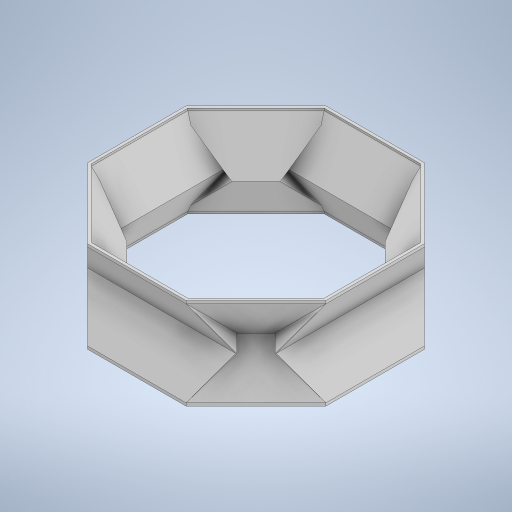
# Autodesk Inventor part: 팔각형 OV-PAM 층 한개
Saved by Autodesk Inventor 2024 (Build 280153000, 153)
## iProperties
Created: 2023-06-16
Part Number: 팔각형 OV-PAM 층 한개
Material: 일반
Document SubType Name: Modeling
Designer: jsw
Density: 1 g/cm^3
Appearance: 기본값
Author: jsw
Autodesk Inventor part; units mm, degrees
ref_plane "YZ Plane" through (0, 0, 0) normal (1, 0, 0) x (0, 1, 0)
ref_plane "XZ Plane" through (0, 0, 0) normal (0, 1, 0) x (-1, 0, 0)
ref_plane "XY Plane" through (0, 0, 0) normal (0, 0, 1) x (1, 0, 0)
sketch "스케치1" plane through (0, 0, 0) normal (0, 1, 0) x (-1, 0, 0)
  line L0 (-32.591883, 13.5) -> (-13.5, 32.591883)
  line L1 (-13.5, 32.591883) -> (13.5, 32.591883)
  line L2 (13.5, 32.591883) -> (32.591883, 13.5)
  line L3 (32.591883, 13.5) -> (32.591883, -13.5)
  line L4 (32.591883, -13.5) -> (13.5, -32.591883)
  line L5 (13.5, -32.591883) -> (-13.5, -32.591883)
  line L6 (-13.5, -32.591883) -> (-32.591883, -13.5)
  line L7 (-32.591883, -13.5) -> (-32.591883, 13.5)
  line L8 (-13.831371, 33.391883) -> (13.831371, 33.391883)
  line L9 (13.831371, 33.391883) -> (33.391883, 13.831371)
  line L10 (33.391883, 13.831371) -> (33.391883, -13.831371)
  line L11 (33.391883, -13.831371) -> (13.831371, -33.391883)
  line L12 (13.831371, -33.391883) -> (-13.831371, -33.391883)
  line L13 (-13.831371, -33.391883) -> (-33.391883, -13.831371)
  line L14 (-33.391883, -13.831371) -> (-33.391883, 13.831371)
  line L15 (-33.391883, 13.831371) -> (-13.831371, 33.391883)
  point P0 (0, 0)
  point P1 (0, 0)
  point P2 (0, 0)
  dimension "d0" = 27
  dimension "d2" = 0.8
  constraints: 32 end point, 2 coincident, 2 horizontal, 34 other
  measures "d0" distance of L0.end L1.end
  measures "d2" distance between parallel lines of L10 L3
extrude "돌출2" add sketch "스케치1" along normal blind 12 contours L0 L1 L2 L3 L4 L5 L6 L7 | L8 L9 L10 L11 L12 L13 L14 L15
ref_plane "작업 평면2" through (33.391883, 0, 13.831371) normal (-0.8660254, -0.5, 0) x (0, 0, -1)
sketch "스케치3" plane through (33.391883, 0, 13.831371) normal (1, 0, 0) x (0, 0, -1)
  line L0 (0, 0) -> (0, 12)
  line L1 (0, 12) -> (27.662742, 12)
  line L2 (0, 0) -> (27.662742, 0)
  line L3 (27.662742, 0) -> (27.662742, 12)
  line L4 (27.662742, 12) -> (0, 12)
  line L5 (0, 12) -> (0, 0)
  line L6 (0, 12) -> (-7.119414, 12)
  line L7 (-19.560512, 12) -> (0, 12)
  line L8 (0, 0) -> (-7.119414, 12)
  line L9 (27.662742, 12) -> (34.782156, 12)
  line L10 (34.782156, 12) -> (27.662742, 0)
  point P0 (13.831371, 0)
  dimension "d17" = 120.68
  dimension "d18" = 120.68
  constraints: 16 end point, 2 parallel, 2 point on line, 1 horizontal, 1 perpendicular
  measures "d17" angle of L8 L2
  measures "d18" angle of L2 L10
extrude "돌출4" cut sketch "스케치3" against normal up to surface surface through (33.391883, 0, 13.831371) normal (-0.8660254, -0.5, 0)
sketch "스케치4" plane through (13.831371, 0, 33.391883) normal (0.7071068, 0, 0.7071068) x (0.7071068, 0, -0.7071068)
  line L0 (0, 0) -> (0, 12)
  line L1 (27.662742, 0) -> (27.662742, 12)
  line L2 (0, 0) -> (27.662742, 0)
  line L3 (27.662742, 0) -> (27.662742, 12)
  line L4 (27.662742, 12) -> (0, 12)
  line L5 (0, 12) -> (0, 0)
  line L6 (27.662742, 0) -> (17.864783, 12)
  line L7 (27.662742, 0) -> (17.593546, 12)
  line L8 (27.662742, 0) -> (0, 0)
  line L9 (0, 0) -> (10.069196, 12)
  line L10 (27.662742, 12) -> (0, 12)
  point P0 (13.831371, 0)
  point P1 (27.662742, 0)
  dimension "d15" = 50
  dimension "d16" = 50
  constraints: 12 end point, 2 parallel, 2 point on line, 1 horizontal, 1 perpendicular
  measures "d15" angle of L7 L4
  measures "d16" angle of L4 L9
ref_plane "작업 평면3" through (13.831371, 0, 33.391883) normal (0.6123724, 0.5, 0.6123724) x (0.7071068, 0, -0.7071068)
extrude "돌출5" cut sketch "스케치4" against normal up to surface contours L9 L4 L7 L2 surface through (13.831371, 0, 33.391883) normal (0.6123724, 0.5, 0.6123724)
pattern_circular "원형 패턴1" count 4 over 360 about axis through (0, -10, 0) along (0, 1, 0) of "돌출4"
pattern_circular "원형 패턴2" count 4 over 360 about axis through (0, -10, 0) along (0, 1, 0) of "돌출5"
mirror "미러5" about plane through (0, 12, 0) normal (0, 1, 0) of "돌출2", "돌출5", "원형 패턴2", "돌출4", "원형 패턴1"
ref_plane "작업 평면5" through (-13.831371, 12, -33.391883) normal (0, 1, 0) x (1, 0, 0)
sketch "스케치9" plane through (-13.831371, 24, -33.391883) normal (0, 1, 0) x (1, 0, 0)
  line L0 (47.223254, -47.223254) -> (47.223254, -19.560512)
  line L1 (47.223254, -19.560512) -> (27.662742, 0)
  line L2 (27.662742, 0) -> (0, 0)
  line L3 (0, 0) -> (-19.560512, -19.560512)
  line L4 (-19.560512, -19.560512) -> (-19.560512, -47.223254)
  line L5 (-19.560512, -47.223254) -> (0, -66.783766)
  line L6 (0, -66.783766) -> (27.662742, -66.783766)
  line L7 (27.662742, -66.783766) -> (47.223254, -47.223254)
  point P0 (13.831371, -33.391883)
extrude "돌출8" add sketch "스케치9" along normal blind 0.8
mirror "미러7" about plane through (-13.831371, 12, -33.391883) normal (0, 1, 0) of "돌출8"
shell "쉘5" thickness 0.8 removed faces 2 at (4.610457, 24.8, 11.130628) at (4.610457, -0.8, 11.130628)
